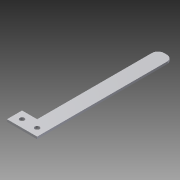
# Autodesk Inventor part: Fork 1 right ver2c
Saved by Autodesk Inventor 2015 (Build 190159000, 159)
## iProperties
Created: 2015-06-20
Part Number: Fork 1 right ver2c
Material: アルミニウム 5052 H32
Document SubType Name: Modeling
Designer: kenta
Density: 2.68 g/cm^3
Appearance: サテン
Mass: 3.99201 g
Surface Area: 23.4464 cm^2
Volume: 1.48956 cm^3
Author: kenta
Autodesk Inventor part; units mm, degrees
ref_plane "YZ Plane" through (0, 0, 0) normal (1, 0, 0) x (0, 1, 0)
ref_plane "XZ Plane" through (0, 0, 0) normal (0, 1, 0) x (-1, 0, 0)
ref_plane "XY Plane" through (0, 0, 0) normal (0, 0, 1) x (1, 0, 0)
sketch "スケッチ1" plane through (0, 0, 0) normal (0, 0, 1) x (1, 0, 0)
  line L0 (0, 0) -> (10, 0)
  line L1 (10, 0) -> (10, -80)
  line L2 (10, -80) -> (0, -80)
  line L3 (0, -80) -> (0, 0)
  dimension "d0" = 10
  dimension "d1" = 80
  constraints: 8 end point, 2 parallel, 1 horizontal, 1 perpendicular
  measures "d0" distance of L1.end L2.end
  measures "d1" distance of L0.end L1.end
extrude "押し出し1" add sketch "スケッチ1" along normal blind 1.5
fillet "フィレット1" radius 4 2 edges at (10, 0, 0.75) (0, 0, 0.75)
sketch "スケッチ2" plane through (0, -80, 0) normal (0, -1, 0) x (1, 0, 0)
  line L0 (-10, 0) -> (10, 0)
  line L1 (10, 0) -> (10, 1.5)
  line L2 (10, 1.5) -> (-10, 1.5)
  line L3 (-10, 1.5) -> (-10, 0)
  line L4 (10, 0) -> (10, 1.5) projected
  line L5 (10, 0) -> (0, 0) projected
  dimension "d35" = 20
  dimension "d36" = 1.5
  dimension "d37" = 0
  dimension "d38" = 0
  constraints: 8 end point, 2 parallel, 1 horizontal, 1 perpendicular
  measures "d35" distance of L2.end L1.end
  measures "d36" distance of L1.end L0.end
  measures "d37" distance between parallel lines of L1 L4
  measures "d38" distance between parallel lines of L5 L0
extrude "押し出し2" add sketch "スケッチ2" along normal blind 10
sketch "スケッチ9" plane through (0, 0, 1.5) normal (0, 0, 1) x (1, 0, 0)
  line L0 (10, -90) -> (-10, -90) projected
  line L1 (10, -4) -> (10, -90) projected
  point P0 (0, 0)
  point P1 (-5, -85)
  point P2 (5, -85)
  dimension "d39" = 10
  dimension "d40" = 5
  dimension "d41" = 5
  constraints: 1 horizontal alignment
  measures "d39" distance of point (5, -85) point (-5, -85)
  measures "d40" distance from line of L0 point (5, -85)
  measures "d41" distance from line of point (5, -85) L1
hole "穴2" at (-5, -85, 1.5) at (5, -85, 1.5) direction (0, 0, -1) diameter 3.1 end through all
